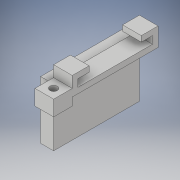
# Autodesk Inventor part: 000.702 - Активный прижим
Saved by Autodesk Inventor 2019 (Build 230136000, 136)
## iProperties
Created: 2020-02-29
Part Number: 000.702 - Активный прижим
Material: Типовые
Document SubType Name: Modeling
Designer: Петров Иван
Density: 1 g/cm^3
Appearance: По умолчанию
Author: Петров Иван
Autodesk Inventor part; units mm, degrees
ref_plane "YZ Plane" through (0, 0, 0) normal (1, 0, 0) x (0, 1, 0)
ref_plane "XZ Plane" through (0, 0, 0) normal (0, 1, 0) x (-1, 0, 0)
ref_plane "XY Plane" through (0, 0, 0) normal (0, 0, 1) x (1, 0, 0)
sketch "Эскиз1" plane through (0, 0, 0) normal (1, 0, 0) x (0, 1, 0)
  line L0 (-2, 20) -> (2, 20)
  line L1 (2, 20) -> (2, -20)
  line L2 (2, -20) -> (-2, -20)
  line L3 (-2, -20) -> (-2, 20)
  line L4 (-2, 20) -> (2, -20) construction
  line L5 (2, 20) -> (-2, -20) construction
  line L6 (2, 20) -> (5, 20)
  line L7 (5, 20) -> (5, 14)
  line L8 (5, 14) -> (2, 14)
  line L9 (2, 14) -> (2, 20)
  line L10 (2, -20) -> (5, -20)
  line L11 (5, -20) -> (5, -14)
  line L12 (5, -14) -> (2, -14)
  line L13 (2, -14) -> (2, -20)
  line L14 (5, 20) -> (-5, 20)
  line L15 (-5, 20) -> (-5, 23)
  line L16 (-5, 23) -> (5, 23)
  line L17 (5, 23) -> (5, 20)
  line L18 (5, -20) -> (-5, -20)
  line L19 (-5, -20) -> (-5, -23)
  line L20 (-5, -23) -> (5, -23)
  line L21 (5, -23) -> (5, -20)
  line L22 (-5, 23) -> (-2, 23)
  line L23 (-2, 23) -> (-2, -23)
  line L24 (-2, -23) -> (-5, -23)
  line L25 (-5, -23) -> (-5, 23)
  point P0 (0, 0)
  dimension "d0" = 4
  dimension "d1" = 40
  dimension "d2" = 3
  dimension "d3" = 6
  dimension "d4" = 3
  dimension "d5" = 6
  dimension "d6" = 10
  dimension "d7" = 10
  dimension "d8" = 3
  dimension "d9" = 3
  constraints: 52 end point, 12 parallel, 6 horizontal, 6 perpendicular, 2 midpoint, 2 point on line
  measures "d0" distance of L1.end L2.end
  measures "d1" distance of L0.end L1.end
  measures "d2" distance of L7.end L8.end
  measures "d3" distance of L6.end L7.end
  measures "d4" distance of L12.end L11.end
  measures "d5" distance of L11.end L10.end
  measures "d6" distance of L15.end L16.end
  measures "d7" distance of L20.end L19.end
  measures "d8" distance of L19.end L18.end
  measures "d9" distance of L16.end L6.end
extrude "Выдавливание1" add sketch "Эскиз1" along normal blind 10 contours L23 L16 L17 L6 L0 | L3 L18 L25 L14 | L14 L15 L16 L23 | L6 L7 L8 L1 | L23 L20 L19 L18 | L2 L10 L21 L20 L23 | L1 L12 L11 L10
sketch "Эскиз2" plane through (0, -5, -23) normal (0, -1, 0) x (1, 0, 0)
  line L0 (10, 37) -> (10, 46) projected
  line L1 (10, 46) -> (0, 46)
  line L2 (0, 46) -> (0, 56)
  line L3 (0, 56) -> (10, 56)
  line L4 (10, 56) -> (10, 46)
  circle A0 centre (5, 51) radius 2
  point P0 (0, 23)
  dimension "d14" = 10
  dimension "d15" = 10
  dimension "d16" = 4
  constraints: 8 end point, 2 parallel, 1 centre point, 1 horizontal, 1 perpendicular
  measures "d14" distance of L2.end L3.end
  measures "d15" distance of L1.end L2.end
  measures "d16" diameter of A0
extrude "Выдавливание2" add sketch "Эскиз2" against normal blind 4 and the other way blind 4.25
sketch "Эскиз3" plane through (0, -5, -23) normal (0, -1, 0) x (1, 0, 0)
  line L0 (0, 46) -> (10, 46) projected
  line L1 (0, 46) -> (-7, 46)
  line L2 (-7, 46) -> (-7, 0)
  line L3 (-7, 0) -> (0, 0)
  line L4 (0, 0) -> (0, 46)
  point P0 (0, 23)
  dimension "d21" = 7
  constraints: 8 end point, 2 parallel, 1 horizontal, 1 perpendicular
  measures "d21" distance of L3.end L2.end
extrude "Выдавливание3" add sketch "Эскиз3" along normal blind 30 and the other way blind 1
chamfer "Фаска1" distance 2 angle 45 1 edges at (0, -4, 0)
